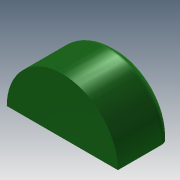
# Autodesk Inventor part: ball socket
Saved by Autodesk Inventor 2015 (Build 190159000, 159)
## iProperties
Created: 2017-05-09
Part Number: ball socket
Material: 일반
Document SubType Name: Modeling
Designer: gatew
Density: 1 g/cm^3
Appearance: 기본값
Author: gatew
Autodesk Inventor part; units mm, degrees
sketch "스케치1" plane through (0, 0, 0) normal (0, 0, 1) x (1, 0, 0)
  arc A0 (0, -7.65) -> (5.8602, 4.9173) centre (0, 0) ccw
  line L0 (0, -7.65) -> (0, -8.65)
  line L1 (0, -8.65) -> (13.6, -8.65)
  line L2 (13.6, -8.65) -> (13.6, 4.8843)
  line L3 (0, 0) -> (7.5, 0) construction
  line L4 (8.5089, 4.8843) -> (13.6, 4.8843)
  line L5 (0, 0) -> (0, 6.3672)
  line L6 (8.5089, 4.8843) -> (6.9333, 3.233)
  dimension "d0" = 15.3
  dimension "d1" = 1
  dimension "d2" = 13.6
  constraints: 14 end point, 3 perpendicular, 3 point on circle, 2 vertical, 1 centre point, 1 coincident, 1 horizontal
  measures "d0" diameter of A0
  measures "d1" distance of L0.start L0.end
  measures "d2" distance of L0.end L1.end
revolve "회전1" add sketch "스케치1" angle 180 about axis through (0, 0, 0) along (0, -1, 0)
sketch "스케치3" plane through (0, 0, 0) normal (0, 0, 1) x (1, 0, 0)
  circle A0 centre (0, 0) radius 2
  dimension "d8" = 4
  constraints: 1 centre point, 1 coincident
  measures "d8" diameter of A0
extrude "돌출2" cut sketch "스케치3" along normal mid plane 12
sketch "스케치4" plane through (0, 0, 0) normal (0, 0, 1) x (1, 0, 0)
  point P0 (0, 0)
  point P1 (0, 0)
  constraints: 1 coincident
sketch "스케치6" plane through (0, 0, 0) normal (0, 0, 1) x (1, 0, 0)
  point P0 (0, 0)
  point P1 (0, 0)
  constraints: 1 coincident
ref_plane "작업 평면1" through (13.6, 4.8843, 7.5) normal (0, 0, -1) x (-1, 0, 0)
ref_plane "작업 평면2" through (13.6, 4.8843, 7.5) normal (0, 0, -1) x (-1, 0, 0)
chamfer "모따기1" distance 2 angle 45 1 edges at (0, 4.8843, 13.6)
ref_plane "작업 평면3" through (0, -1.8829, 13.6) normal (0, 0, -1) x (-1, 0, 0)
ref_plane "작업 평면4" through (0, 0, 7.5) normal (0, 0, -1) x (-1, 0, 0)
fillet "모깎기2" radius 2 2 edges at (0, 2.8843, 13.6) (0, 4.8843, 11.6)
